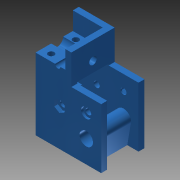
# Autodesk Inventor part: YIdlerBlockLeft.old
Saved by Autodesk Inventor 2015 (Build 190159000, 159)
## iProperties
Created: 2014-08-14
Part Number: YIdlerBlockLeft.old
Material: ABS Plastic
Document SubType Name: Modeling
Designer: t_clevj
Density: 1.06 g/cm^3
Appearance: Cyan
Author: t_clevj
Autodesk Inventor part; units mm, degrees
ref_plane "YZ Plane" through (0, 0, 0) normal (1, 0, 0) x (0, 1, 0)
ref_plane "XZ Plane" through (0, 0, 0) normal (0, 1, 0) x (-1, 0, 0)
ref_plane "XY Plane" through (0, 0, 0) normal (0, 0, 1) x (1, 0, 0)
sketch "Sketch1" plane through (0, 0, 0) normal (0, 1, 0) x (-1, 0, 0)
  line L0 (0, 0) -> (44, 0)
  line L1 (44, 0) -> (44, 60)
  line L2 (44, 60) -> (20, 60)
  line L3 (20, 60) -> (20, 40)
  line L4 (20, 40) -> (0, 40)
  line L5 (0, 40) -> (0, 0)
  dimension "d0" = 44
  dimension "d1" = 60
  dimension "d2" = 24
  dimension "d3" = 20
  constraints: 12 end point, 4 perpendicular, 2 horizontal
  measures "d0" distance of L0.start L0.end
  measures "d1" distance of L0.end L1.end
  measures "d2" distance of L1.end L2.end
  measures "d3" distance of L2.end L3.end
extrude "BaseBottom" add sketch "Sketch1" along normal blind 4
sketch "Sketch2" plane through (0, 4, 0) normal (0, 1, 0) x (1, 0, 0)
  line L0 (0, 0) -> (-44, 0) projected
  line L1 (-44, 0) -> (-44, -60) projected
  line L2 (-44, -60) -> (-20, -60) projected
  line L3 (-20, -60) -> (-20, -40) projected
  line L4 (-20, -40) -> (0, -40) projected
  line L5 (0, -40) -> (0, 0) projected
  circle A0 centre (-10, -15) radius 5
  line L6 (-5.072, -14.1547) -> (-7.5, 0)
  line L7 (-14.928, -14.1547) -> (-12.5, 0)
  line L8 (-20, -41) -> (-44, -41)
  arc A1 (-34, -15.7805) -> (-37.798, -20) centre (-28, -25) ccw
  line L9 (-34, 0) -> (-34, -15.7805)
  line L10 (-37.798, -20) -> (-44, -20)
  dimension "d6" = 10
  dimension "d7" = 10
  dimension "d8" = 15
  dimension "d9" = 5
  dimension "d10" = 7.5
  dimension "d11" = 1
  dimension "d12" = 22
  dimension "d13" = 25
  dimension "d14" = 16
  dimension "d15" = 10
  dimension "d16" = 20
  constraints: 10 end point, 6 point on line, 4 point on circle, 2 centre point, 2 perpendicular, 2 tangent, 1 vertical
  measures "d6" diameter of A0
  measures "d7" distance from line of L5 A0.centre
  measures "d8" distance from line of L0 A0.centre
  measures "d9" distance of L6.end L7.end
  measures "d10" distance from line of L5 L6.end
  measures "d11" distance between parallel lines of L4 L8
  measures "d12" diameter of A1
  measures "d13" distance from line of L0 A1.centre
  measures "d14" distance from line of L1 A1.centre
  measures "d15" distance between parallel lines of L1 L9
  measures "d16" distance between parallel lines of L0 L10
extrude "SpannerMaterial" add sketch "Sketch2" along normal blind 21 contours L6 A0 L7 L0 | A0 | L9 A1 L10 L1 L0 | L3 L2 L1 L8
sketch "Sketch3" plane through (0, 25, 0) normal (0, 1, 0) x (1, 0, 0)
  line L0 (-34, 0) -> (-44, 0) projected
  line L1 (-34, 0) -> (0, 0)
  line L2 (0, 0) -> (0, -40)
  line L3 (0, -40) -> (-20, -40)
  line L4 (-20, -40) -> (-20, -60)
  line L5 (-20, -60) -> (-44, -60)
  line L6 (-44, -60) -> (-44, 0)
  constraints: 12 end point, 5 perpendicular, 1 horizontal
extrude "TopSurface" add sketch "Sketch3" along normal blind 4
sketch "Sketch4" plane through (-44, 0, 0) normal (-1, 0, 0) x (0, 0, 1)
  line L0 (0, 0) -> (60, 0) projected
  line L1 (60, 0) -> (60, 29) projected
  line L2 (60, 25) -> (48, 25)
  line L3 (48, 25) -> (48, 0)
  dimension "d21" = 12
  dimension "d22" = 25
  constraints: 4 end point, 2 point on line, 1 horizontal, 1 perpendicular
  measures "d21" distance of L2.start L2.end
  measures "d22" distance of L2.end L3.end
extrude "YRodNotch" cut sketch "Sketch4" against normal blind 20
sketch "Sketch6" plane through (-44, 0, 0) normal (-1, 0, 0) x (0, 0, 1)
  line L0 (48, 25) -> (60, 25) projected
  line L1 (48, 0) -> (48, 25) projected
  circle A0 centre (48, 14.5) radius 4
  dimension "d29" = 8
  dimension "d30" = 10.5
  constraints: 1 centre point, 1 point on line
  measures "d29" diameter of A0
  measures "d30" distance from line of L0 A0.centre
extrude "YRodHole" cut sketch "Sketch6" against normal up to surface (20 mm away)
sketch "YRodClampSketch" plane through (-44, 25, 48) normal (0, 0, 1) x (1, 0, 0)
  line L0 (20, -14.5) -> (0, -14.5) projected
  line L1 (0, -25) -> (0, -14.5) projected
  line L2 (20, -25) -> (0, -25) projected
  line L3 (20, -25) -> (20, -14.5) projected
  circle A0 centre (6, -4) radius 2
  circle A1 centre (6, -20.5) radius 2
  line L4 (0, -6.5) -> (0, 0) projected
  point P0 (44, -25)
  dimension "d33" = 4
  dimension "d34" = 4
  dimension "d76" = 6
  dimension "d118" = 4.5
  dimension "d119" = 21
  constraints: 2 centre point, 1 vertical alignment
  measures "d33" diameter of A0
  measures "d34" diameter of A1
  measures "d76" distance from line of L4 A0.centre
  measures "d118" distance from line of L2 A1.centre
  measures "d119" distance from line of L2 A0.centre
extrude "YRodClampHoles" cut sketch "YRodClampSketch" against normal up to surface (7 mm away) contours A0 | A1
sketch "Sketch10" plane through (-20, 25, 41) normal (0, 0, -1) x (-1, 0, 0)
  arc A0 (19.9365, -21) -> (16.0635, -21) centre (18, -20.5) ccw projected
  circle A1 centre (18, -4) radius 2 projected
  line L0 (22.0415, -4) -> (20.0207, -7.5)
  line L1 (20.0207, -7.5) -> (15.9793, -7.5)
  line L2 (15.9793, -7.5) -> (13.9585, -4)
  line L3 (13.9585, -4) -> (15.9793, -0.5)
  line L4 (15.9793, -0.5) -> (20.0207, -0.5)
  line L5 (20.0207, -0.5) -> (22.0415, -4)
  line L6 (22.0415, -20.5) -> (20.0207, -24)
  line L7 (20.0207, -24) -> (15.9793, -24)
  line L8 (15.9793, -24) -> (13.9585, -20.5)
  line L9 (13.9585, -20.5) -> (15.9793, -17)
  line L10 (15.9793, -17) -> (20.0207, -17)
  line L11 (20.0207, -17) -> (22.0415, -20.5)
  point P0 (-20, -25)
  point P1 (18, -4)
  point P2 (18, -20.5)
  dimension "d46" = 7
  constraints: 24 end point, 2 coincident, 2 horizontal, 1 parallel, 26 other
  measures "d46" distance between parallel lines of L10 L7
extrude "YRodClampNutTraps" cut sketch "Sketch10" along normal blind 4 and the other way blind 4
sketch "Sketch11" plane through (-44, 25, 48) normal (0, -1, 0) x (1, 0, 0)
  line L0 (0, 0) -> (20, 0) projected
  circle A0 centre (14.9, 0) radius 2.5
  line L1 (20, 0) -> (20, 12) projected
  point P0 (44, -48)
  dimension "d51" = 5
  dimension "d77" = 5.1
  constraints: 1 centre point, 1 point on line
  measures "d51" diameter of A0
  measures "d77" distance from line of L1 A0.centre
extrude "FrameBoltHoleYRodTop" cut sketch "Sketch11" against normal up to surface (4 mm away)
sketch "Sketch15" plane through (-24, 0, 0) normal (-1, 0, 0) x (0, 0, 1)
  arc A0 (48, 18.5) -> (48, 10.5) centre (48, 14.5) ccw projected
  circle A1 centre (48, 14.5) radius 2.5
  point P0 (0, 0)
  dimension "d64" = 5
  constraints: 1 centre point, 1 coincident
  measures "d64" diameter of A1
extrude "FrameBoltHoleYRodSide" cut sketch "Sketch15" against normal up to surface (4 mm away)
ref_plane "Work Plane1" through (-44, 29, 50) normal (0, 0, 1) x (1, 0, 0)
sketch "Sketch18" plane through (-44, 18.5, 48) normal (0, 0, 1) x (1, 0, 0)
  line L0 (0, 6.5) -> (12.4, 6.5) projected
  line L1 (9.8, 6.5) -> (12.4, 10.1)
  line L2 (12.4, 10.1) -> (12.4, 6.5)
  line L3 (17.4, 6.5) -> (12.4, 6.5) projected
  line L4 (12.4, 6.5) -> (9.8, 6.5)
  line L5 (14.9, 6.5) -> (14.9, 10.5128)
  point P0 (44, -18.5)
  dimension "d78" = 2.6
  dimension "d79" = 3.6
  constraints: 8 end point, 1 collinear, 1 midpoint, 1 perpendicular, 1 point on line, 1 vertical
  measures "d78" distance from line of L1.start L2
  measures "d79" distance of L1.end L0.end
revolve "FrameBoltChamferYRodTop" cut sketch "Sketch18" angle 360 about axis through (-29.1, 25, 48) along (0, 1, 0)
sketch "Sketch21" plane through (0, 0, 0) normal (0, -1, 0) x (1, 0, 0)
  arc A0 (-5.072, 14.1547) -> (-14.928, 14.1547) centre (-10, 15) ccw projected
  arc A1 (-5.072, 14.1547) -> (-14.928, 14.1547) centre (-10, 15) ccw projected
hole "FrameBoltBackTop" at (-10, 0, 15) direction (0, 1, 0) diameter 5 end up to face face through (-21.3333, 29, 13.3333) facing (0, 1, 0) counterbore diameter 9 counterbore depth 25
sketch "Sketch22" plane through (0, 29, 0) normal (0, 1, 0) x (1, 0, 0)
  line L0 (-44, 0) -> (-44, -60) projected
  line L1 (0, 0) -> (-44, 0) projected
  point P0 (-28, -25)
  dimension "d94" = 25
  dimension "d95" = 16
  measures "d94" distance from line of L1 point (-28, -25)
  measures "d95" distance from line of L0 point (-28, -25)
hole "BearingHoleInner" at (-28, 29, 25) direction (0, -1, 0) diameter 4 end up to face face through (-36, 0, 29.3333) facing (0, -1, 0) counterbore diameter 7 counterbore depth 1.5
sketch "Sketch23" plane through (0, 0, 0) normal (0, -1, 0) x (1, 0, 0)
  line L0 (0, 0) -> (-44, 0) projected
  line L1 (0, 40) -> (0, 0) projected
  point P0 (-10, 30)
  dimension "d103" = 30
  dimension "d104" = 10
  measures "d103" distance from line of L0 point (-10, 30)
  measures "d104" distance from line of L1 point (-10, 30)
hole "BearingHoleOuter" at (-10, 0, 30) direction (0, 1, 0) diameter 4 end up to face face through (-39.8333, 29, 28.3333) facing (0, 1, 0) counterbore diameter 7 counterbore depth 1.5
sketch "Sketch24" plane through (0, 29, 0) normal (0, 1, 0) x (1, 0, 0)
  circle A0 centre (-10, -30) radius 2 projected
  line L0 (-10, -34.0415) -> (-13.5, -32.0207)
  line L1 (-13.5, -32.0207) -> (-13.5, -27.9793)
  line L2 (-13.5, -27.9793) -> (-10, -25.9585)
  line L3 (-10, -25.9585) -> (-6.5, -27.9793)
  line L4 (-6.5, -27.9793) -> (-6.5, -32.0207)
  line L5 (-6.5, -32.0207) -> (-10, -34.0415)
  dimension "d112" = 7
  constraints: 12 end point, 1 coincident, 1 vertical, 13 other
  measures "d112" distance between parallel lines of L1 L4
extrude "BearingHoleOuterNutTrap" cut sketch "Sketch24" against normal blind 3.2
sketch "Sketch25" plane through (0, 0, 0) normal (0, -1, 0) x (1, 0, 0)
  circle A0 centre (-28, 25) radius 2 projected
  line L0 (-28, 29.0415) -> (-24.5, 27.0207)
  line L1 (-24.5, 27.0207) -> (-24.5, 22.9793)
  line L2 (-24.5, 22.9793) -> (-28, 20.9585)
  line L3 (-28, 20.9585) -> (-31.5, 22.9793)
  line L4 (-31.5, 22.9793) -> (-31.5, 27.0207)
  line L5 (-31.5, 27.0207) -> (-28, 29.0415)
  dimension "d115" = 7
  constraints: 12 end point, 1 coincident, 1 vertical, 13 other
  measures "d115" distance between parallel lines of L1 L4
extrude "BearingHoleInnerNutTrap" cut sketch "Sketch25" against normal blind 2.5
sketch "Sketch26" plane through (0, 0, 0) normal (0, -1, 0) x (1, 0, 0)
  circle A0 centre (-29.1, 48) radius 2.5 projected
  circle A1 centre (-29.1, 48) radius 1.8
  dimension "d120" = 3.6
  constraints: 1 centre point, 1 coincident
  measures "d120" diameter of A1
extrude "Extrusion20" cut sketch "Sketch26" against normal up to surface (29 mm away) contours A1
sketch "Sketch27" plane through (-44, 25, 48) normal (0, 1, 0) x (1, 0, 0)
  arc A0 (16.7, 0) -> (13.1, 0) centre (14.9, 0) ccw projected
  line L0 (16.7, 0) -> (20, 0) projected
  line L1 (20, 0) -> (20, -1.005) projected
  arc A1 (20, 0) -> (9.8, 0) centre (14.9, 0) ccw projected
  line L2 (9.8, 0) -> (13.1, 0) projected
  point P0 (44, 48)
  point P1 (19.6, 0)
  constraints: 1 other
extrude "Extrusion21" cut sketch "Sketch27" against normal blind 6
body "Solid1"
